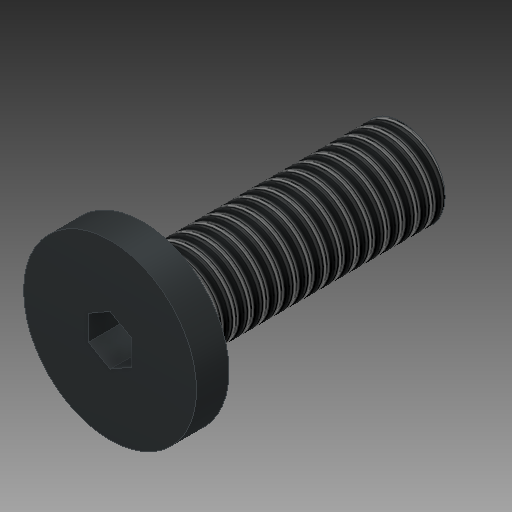
# Autodesk Inventor part: M4極低頭ネジ　12
Saved by Autodesk Inventor 2017.3 (Build 213256000, 256)
## iProperties
Part Number: M4極低頭ネジ　12
Material: 鋼、高強度、低合金
Document SubType Name: Modeling
Designer: 原知也
Density: 7.85 g/cm^3
Appearance: 鉄 灰色
Mass: 1.70765 g
Surface Area: 3.06347 cm^2
Volume: 0.217534 cm^3
Author: 原知也
Autodesk Inventor part; units mm, degrees
ref_plane "YZ Plane" through (0, 0, 0) normal (1, 0, 0) x (0, 1, 0)
ref_plane "XZ Plane" through (0, 0, 0) normal (0, 1, 0) x (-1, 0, 0)
ref_plane "XY Plane" through (0, 0, 0) normal (0, 0, 1) x (1, 0, 0)
sketch "スケッチ1" plane through (0, 0, 0) normal (0, 0, 1) x (1, 0, 0)
  circle A0 centre (0, 0) radius 2
  dimension "d0" = 4
  constraints: 1 centre point, 1 coincident
  measures "d0" diameter of A0
extrude "押し出し1" add sketch "スケッチ1" along normal blind 12
thread "ねじ1" size "M4x0.7" class "6g" standard "ANSI Metric M Profile" full length
sketch "スケッチ2" plane through (0, 0, 12) normal (0, 0, 1) x (1, 0, 0)
  circle A0 centre (0, 0) radius 4
  dimension "d5" = 8
  constraints: 1 centre point, 1 coincident
  measures "d5" diameter of A0
extrude "押し出し2" add sketch "スケッチ2" along normal blind 1.5
sketch "スケッチ3" plane through (0, 0, 13.5) normal (0, 0, 1) x (1, 0, 0)
  line L0 (0, 1.1547) -> (1, 0.5774)
  line L1 (1, 0.5774) -> (1, -0.5774)
  line L2 (1, -0.5774) -> (0, -1.1547)
  line L3 (0, -1.1547) -> (-1, -0.5774)
  line L4 (-1, -0.5774) -> (-1, 0.5774)
  line L5 (-1, 0.5774) -> (0, 1.1547)
  point P0 (0, 0)
  point P1 (0, 0)
  dimension "d8" = 2
  constraints: 12 end point, 1 coincident, 13 other
  measures "d8" distance between parallel lines of L1 L4
extrude "押し出し3" cut sketch "スケッチ3" against normal blind 2.5
